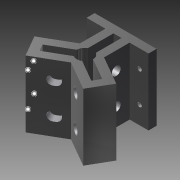
# Autodesk Inventor part: LinearBearing
Saved by Autodesk Inventor 2011 (Build 150239000, 239)
## iProperties
Created: 2010-04-15
Part Number: LinearBearing
Document SubType Name: Modeling
Designer: James Taylor
Density: 1 g/cm^3
Mass: 96.3722 g
Surface Area: 330.214 cm^2
Volume: 96.3722 cm^3
LegAngle: 120.00 deg
BearingWidth: 7.000 mm
BearingPadding: 0.200 mm
BearingOuterDiameter: 22.000 mm
Author: James Taylor
Autodesk Inventor part; units mm, degrees
ref_plane "YZ Plane" through (0, 0, 0) normal (1, 0, 0) x (0, 1, 0)
ref_plane "XZ Plane" through (0, 0, 0) normal (0, 1, 0) x (-1, 0, 0)
ref_plane "XY Plane" through (0, 0, 0) normal (0, 0, 1) x (1, 0, 0)
sketch "Sketch - Bearing Body" plane through (0, 0, 0) normal (0, 0, 1) x (1, 0, 0)
  line L0 (55.8, 0) -> (55.8, 7.3)
  line L1 (55.8, 7.3) -> (0, 7.3)
  line L2 (0, 7.3) -> (0, 0)
  line L3 (38.8, 0) -> (38.8, -23)
  line L4 (17, -23) -> (17, 0)
  line L5 (17, -23) -> (-8.9808, -38)
  line L6 (-8.9808, -38) -> (1.9192, -56.8794)
  line L7 (1.9192, -56.8794) -> (27.9, -41.8794)
  line L8 (38.8, -23) -> (64.7808, -38)
  line L9 (64.7808, -38) -> (53.8808, -56.8794)
  line L10 (53.8808, -56.8794) -> (27.9, -41.8794)
  line L11 (0, 0) -> (17, 0)
  line L12 (38.8, 0) -> (55.8, 0)
  line L13 (24.3, 0) -> (31.5, 0)
  line L14 (31.5, 0) -> (31.5, -22.9717)
  line L15 (24.3, -22.9717) -> (24.3, 0)
  line L16 (0.9912, -40.672) -> (4.5912, -46.9074)
  line L17 (4.5912, -46.9074) -> (24.077, -35.6572)
  line L18 (0.9912, -40.672) -> (20.55, -29.3797)
  line L19 (51.2088, -46.9074) -> (54.8088, -40.672)
  line L20 (54.8088, -40.672) -> (35.25, -29.3797)
  line L21 (51.2088, -46.9074) -> (31.723, -35.6572)
  circle A0 centre (27.9, -29.3797) radius 7.35
  point P0 (17, -11.5)
  point P1 (51.7904, -30.5)
  dimension "d1" = 7.3
  dimension "d3" = 23
  dimension "LegLength" = 30
  dimension "d7" = 21.8
  dimension "d12" = 30
  dimension "d13" = 21.8
  dimension "LegAngle2" = 120
  dimension "d15" = 120
  dimension "d17" = 21.8
  dimension "d19" = 17
  dimension "d20" = 17
  dimension "d22" = 7.2
  dimension "d23" = 7.3
  dimension "d24" = 7.3
  dimension "d25" = 7.2
  dimension "d26" = 7.3
  dimension "d27" = 7.2
  dimension "d28" = 7.3
  dimension "d29" = 7.3
  dimension "d77" = 14.7
  constraints: 45 end point, 10 perpendicular, 9 parallel, 6 point on circle, 3 horizontal, 2 collinear, 2 midpoint, 1 centre point, 1 horizontal alignment, 1 vertical, 1 vertical alignment
  measures "d1" distance of L0.end L0.start
  measures "d3" distance of L3.start L3.end
  measures "LegLength" distance of L4.start L5.end
  measures "d7" distance of L5.end L6.end
  measures "d12" distance of L3.end L8.end
  measures "d13" distance of L8.end L9.end
  measures "LegAngle2" angle of L5 L4
  measures "d15" angle of L8 L3
  measures "d17" distance between parallel lines of L3 L4
  measures "d19" distance of L2.end L4.end
  measures "d20" distance of L3.start L0.start
  measures "d22" distance of L13.start L13.end
  measures "d23" distance between parallel lines of L4 L15
  measures "d24" distance between parallel lines of L6 L16
  measures "d25" distance of L16.start L16.end
  measures "d26" distance between parallel lines of L5 L18
  measures "d27" distance of L19.start L19.end
  measures "d28" distance between parallel lines of L10 L21
  measures "d29" distance between parallel lines of L9 L19
  measures "d77" diameter of A0
extrude "Extrusion - Bearing Body" add sketch "Sketch - Bearing Body" along normal blind 60
sketch "Sketch - Bearing Screw Holes 1" plane through (17, -23, 60) normal (-0.5, 0.866, 0) x (0.866, 0.5, 0)
  line L0 (-30, 0) -> (0, 0) projected
  line L1 (-30, 60) -> (0, 60) projected
  line L2 (-30, 60) -> (-30, 0) projected
  line L3 (0, 60) -> (0, 0) projected
  line L4 (-12.1, 48.2) -> (-10.1, 48.2)
  line L5 (-12.1, 39.8) -> (-10.1, 39.8)
  line L6 (-12.1, 20.2) -> (-10.1, 20.2)
  line L7 (-12.1, 11.8) -> (-10.1, 11.8)
  arc A0 (-12.1, 20.2) -> (-12.1, 11.8) centre (-12.1, 16) ccw
  arc A1 (-10.1, 11.8) -> (-10.1, 20.2) centre (-10.1, 16) ccw
  arc A2 (-10.1, 39.8) -> (-10.1, 48.2) centre (-10.1, 44) ccw
  arc A3 (-12.1, 48.2) -> (-12.1, 39.8) centre (-12.1, 44) ccw
  point P0 (-3.2224, 60)
  point P1 (-11.1, 16)
  point P2 (-11.1, 44)
  point P3 (-11.1, 48.2)
  point P4 (-11.1, 39.8)
  point P5 (-11.1, 20.2)
  point P6 (-11.1, 11.8)
  dimension "d47" = 16
  dimension "d48" = 18.9
  dimension "d49" = 16
  dimension "BearingHoleElipseMiddle" = 2
  dimension "BearingBoltRadius" = 4.2
  dimension "d91" = 4.2
  dimension "d92" = 4.2
  dimension "d93" = 4.2
  dimension "d94" = 4.2
  constraints: 8 end point, 8 point on circle, 6 parallel, 5 vertical alignment, 4 centre point, 4 midpoint, 3 equal radius, 1 perpendicular
  measures "d47" distance from line of L1 point (-11.1, 44)
  measures "d48" distance from line of L2 point (-11.1, 44)
  measures "d49" distance from line of L0 point (-11.1, 16)
  measures "BearingHoleElipseMiddle" distance of L4.start L4.end
  measures "BearingBoltRadius" distance from line of L4 point (-11.1, 44)
  measures "d91" distance from line of point (-11.1, 44) L5
  measures "d92" distance from line of point (-11.1, 16) L6
  measures "d93" distance from line of point (-11.1, 16) L7
  measures "d94" radius of A3
sketch "Sketch - Bearing Screw Holes 2" plane through (64.7808, -38, 60) normal (0.5, 0.866, 0) x (0.866, -0.5, 0)
  line L0 (-30, 0) -> (0, 0) projected
  line L1 (0, 60) -> (0, 0) projected
  line L2 (-30, 60) -> (0, 60) projected
  point P0 (-75.1018, 60)
  point P1 (-18.9, 16)
  point P2 (-18.9, 44)
  dimension "d50" = 18.9
  dimension "d51" = 16
  dimension "d52" = 16
  constraints: 1 vertical alignment
  measures "d50" distance from line of L1 point (-18.9, 44)
  measures "d51" distance from line of L2 point (-18.9, 44)
  measures "d52" distance from line of L0 point (-18.9, 16)
hole "Hole - Bearing Screw Holes 2" at (48.4129, -28.55, 16) at (48.4129, -28.55, 44) direction (-0.5, -0.866, 0) diameter 9 end through all clearance for "Socket Head Cap Screw ISO 4762" size "M8" standard "ISO"
sketch "Sketch - Bearing Screw Holes 3" plane through (17, -23, 0) normal (-1, 0, 0) x (0, 0, 1)
  line L0 (60, 0) -> (60, 23) projected
  line L1 (0, 23) -> (60, 23) projected
  line L2 (0, 0) -> (0, 23) projected
  point P0 (16, 10.97)
  point P1 (44, 10.97)
  dimension "d67" = 16
  dimension "d68" = 12.03
  dimension "d69" = 16
  constraints: 1 horizontal alignment
  measures "d67" distance from line of L2 point (16, 10.97)
  measures "d68" distance from line of L1 point (16, 10.97)
  measures "d69" distance from line of L0 point (44, 10.97)
hole "Hole - Bearing Screw Holes 3" at (17, -12.03, 16) at (17, -12.03, 44) direction (1, 0, 0) diameter 8 end through all clearance for "Hex Head Cap Screw ISO 24017" size "M8" standard "ISO"
sketch "Sketch - Plate Holes" plane through (0, 7.3, 0) normal (0, 1, 0) x (1, 0, 0)
  line L0 (0, -60) -> (55.8, -60) projected
  line L1 (55.8, 0) -> (55.8, -60) projected
  line L2 (0, 0) -> (55.8, 0) projected
  line L3 (0, 0) -> (0, -60) projected
  point P0 (8, -16)
  point P1 (8, -44)
  point P2 (47.8, -16)
  point P3 (47.8, -44)
  dimension "PlateAttachmentHoleVert" = 16
  dimension "d79" = 16
  dimension "PlateAttachmentHoleHoriz" = 8
  dimension "d81" = 8
  constraints: 2 horizontal alignment, 2 vertical alignment
  measures "PlateAttachmentHoleVert" distance from line of L2 point (8, -16)
  measures "d79" distance from line of L0 point (8, -44)
  measures "PlateAttachmentHoleHoriz" distance from line of L3 point (8, -16)
  measures "d81" distance from line of L1 point (47.8, -16)
hole "Hole - Plate Holes" at (8, 7.3, 16) at (8, 7.3, 44) at (47.8, 7.3, 16) at (47.8, 7.3, 44) direction (0, -1, 0) diameter 3.797 depth 7.3 tip angle 118 clearance for "Flat Head Machine Screw (82)" size "#6" standard "Ansi Unified Screw Threads"
extrude "Extrusion4" cut sketch "Sketch - Bearing Screw Holes 1" against normal through all contours L4 A2 L5 A3 | L6 A1 L7 A0
sketch "Sketch7" plane through (-8.9808, -38, 0) normal (-0.866, -0.5, 0) x (0, 0, 1)
  line L0 (60, -21.8) -> (60, 0) projected
  line L1 (0, 0) -> (60, 0) projected
  line L2 (0, -21.8) -> (0, 0) projected
  line L3 (0, -21.8) -> (60, -21.8) projected
  point P0 (0, 28.4186)
  point P1 (16, -3.65)
  point P2 (16, -18.15)
  point P3 (44, -18.15)
  point P4 (44, -3.65)
  dimension "d97" = 3.65
  dimension "d98" = 3.65
  dimension "d99" = 16
  dimension "d100" = 16
  constraints: 2 horizontal alignment, 2 vertical alignment
  measures "d97" distance from line of L1 point (16, -3.65)
  measures "d98" distance from line of L3 point (16, -18.15)
  measures "d99" distance from line of L2 point (16, -3.65)
  measures "d100" distance from line of L0 point (44, -3.65)
hole "Hole5" at (-7.1558, -41.161, 16) at (0.0942, -53.7184, 16) at (0.0942, -53.7184, 44) at (-7.1558, -41.161, 44) direction (0.866, 0.5, 0) diameter 2.642 depth 15 thread size "6-32 UNC" class "2B" standard "ANSI Unified Screw Threads"
equation "\"d1\" = WallWidth"
equation "\"d7\" = SupportWidth"
equation "\"d12\" = LegLength"
equation "\"d13\" = SupportWidth"
equation "\"LegAngle2\" = LegAngle"
equation "\"d15\" = LegAngle"
equation "\"d17\" = SupportWidth"
equation "\"d19\" = PlateHangOver"
equation "\"d20\" = PlateHangOver"
equation "\"d22\" = BearingWidth + BearingPadding"
equation "\"d23\" = WallWidth"
equation "\"d24\" = WallWidth"
equation "\"d25\" = BearingWidth + BearingPadding"
equation "\"d26\" = WallWidth"
equation "\"d27\" = BearingWidth + BearingPadding"
equation "\"d28\" = WallWidth"
equation "\"d29\" = WallWidth"
equation "\"d47\" = BearingHorizontalDistance"
equation "\"d48\" = BearingVerticalHoleDistance"
equation "\"d49\" = BearingHorizontalDistance"
equation "\"BearingBoltRadius\" = 0.5 * BearingHoleSize"
equation "\"d91\" = 0.5 * BearingHoleSize"
equation "\"d92\" = 0.5 * BearingHoleSize"
equation "\"d93\" = 0.5 * BearingHoleSize"
equation "\"d94\" = 0.5 * BearingHoleSize"
equation "\"d50\" = BearingVerticalHoleDistance"
equation "\"d51\" = BearingHorizontalDistance"
equation "\"d52\" = BearingHorizontalDistance"
equation "\"d79\" = PlateAttachmentHoleVert"
equation "\"d81\" = PlateAttachmentHoleHoriz"
equation "\"d87\" = WallWidth"
equation "\"d97\" = 0.5 * WallWidth"
equation "\"d98\" = 0.5 * WallWidth"
equation "\"d99\" = BearingHorizontalDistance"
equation "\"d100\" = BearingHorizontalDistance"
equation "\"LegAngle\" = 120deg"
equation "\"BearingWidth\" = 7"
equation "\"BearingOuterDiameter\" = 22"
equation "\"BearingPadding\" = 0.2"
equation "\"SupportWidth\" = BearingWidth + 2 * WallWidth + BearingPadding"
equation "\"PlateHangOver\" = 17"
equation "\"RodDiameter\" = 12.7"
equation "\"RodDiameterPadding\" = 2"
equation "\"WallWidth\" = 7.3"
equation "\"BearingHoleSize\" = 8.4"
equation "\"BearingHorizontalDistance\" = 16"
equation "\"BearingVerticalHoleDistance\" = 18.9"
body "Solid1"
